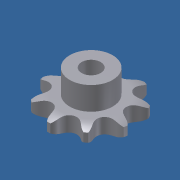
# Autodesk Inventor part: Roller Chain Sprocket1
Saved by Autodesk Inventor 2011 SP1 (Build 150282100, 282)
## iProperties
Created: 2011-02-10
Part Number: Roller Chain Sprocket1
Material: Steel
Document SubType Name: Modeling
Designer: Antonella Wilby
Density: 1 g/cm^3
CustomPartVersion: 1
da_z: 9.0000 ul
da_p: 0.5000 in
da_Dr: 0.3120 in
da_Re: 0.4118 in
da_Ri: 0.1583 in
da_Alfa: 130.00 deg
form_type: 0.0000 ul
da_SC: 0.0023 in
da_Ha: 0.1500 in
da_pt: 0.5660 in
da_k: 1.0000 ul
da_Bf: 0.2962 in
da_Ba: 0.0625 in
da_Rx: 0.5315 in
da_Ra: 0.0200 in
da_Bs: 0.2962 in
da_Ds: 0.8037 in
d42: 0.0000 in
d28: 0.0000 in
d29: 0.0000 in
Author: Antonella Wilby
Autodesk Inventor part; units mm, degrees
ref_plane "YZ Plane" through (0, 0, 0) normal (1, 0, 0) x (0, 1, 0)
ref_plane "XZ Plane" through (0, 0, 0) normal (0, 1, 0) x (-1, 0, 0)
sketch "Theoretical Tooth Profile" plane through (0, 0, 0) normal (0, 0, 1) x (1, 0, 0)
  circle A0 centre (0, 0) radius 18.5662 construction
  line L0 (0, 0) -> (0, 18.5662) construction
  line L1 (0, 0) -> (11.9341, 14.2225) construction
  circle A1 centre (0, 0) radius 21.2565
  arc A2 (-3.0033, 15.8935) -> (3.0033, 15.8935) centre (0, 18.5662) ccw
  line L2 (0, 18.5662) -> (11.9341, 14.2225) construction
  line L3 (0, 18.5662) -> (4.736, 22.7809) construction
  line L4 (4.736, 22.7809) -> (-4.2462, 17.6182) construction
  arc A3 (6.4457, 20.2556) -> (4.5508, 18.1482) centre (10.4256, 14.7715) ccw
  arc A4 (-4.5508, 18.1482) -> (-6.4457, 20.2556) centre (-10.4256, 14.7715) ccw
  line L5 (-10.4256, 14.7715) -> (-4.5508, 18.1482) construction
  arc A5 (-4.2462, 17.6182) -> (-3.0033, 15.8935) centre (4.736, 22.7809) ccw
  line L6 (-4.2462, 17.6182) -> (-4.5508, 18.1482)
  arc A6 (3.0033, 15.8935) -> (4.2462, 17.6182) centre (-4.736, 22.7809) ccw
  line L7 (4.5508, 18.1482) -> (4.2462, 17.6182)
  line L8 (0, 0) -> (7.2701, 19.9746) construction
  point P0 (5.967, 16.3943)
  dimension "d0" = 37.1323
  dimension "d2" = 40
  dimension "d3" = 4.0203
  dimension "d10" = 131.667
  dimension "d11" = 11.778
  dimension "d12" = 6.3398
  dimension "d13" = 10.3602
  dimension "d14" = 11.0947
  dimension "d23" = 3.81
  constraints: 18 end point, 15 point on circle, 7 centre point, 3 coincident, 3 point on line, 3 symmetric about line, 3 tangent, 1 equal radius, 1 midpoint, 1 parallel, 1 vertical, 1 other
  measures "d0" diameter of A0
  measures "d2" angle of L1 L0
  measures "d3" radius of A2
  measures "d10" angle of L3 L0
  measures "d11" angle of L4 L3
  measures "d12" distance of L2.start L3.end
  measures "d13" distance of L3.end L4.end
  measures "d14" distance of A3.centre L0.end
  measures "d23" distance from line of L8.end L2
sketch "Tooth Profile" plane through (0, 0, 0) normal (0, 0, 1) x (1, 0, 0)
  circle A0 centre (0, 0) radius 21.2565 projected
  line L0 (0, 0) -> (0, 18.5662) construction
  line L1 (0, 18.5662) -> (3.6436, 16.8671) construction
  arc A1 (-3.6436, 16.8671) -> (3.6436, 16.8671) centre (0, 18.5662) ccw
  line L2 (-3.6436, 16.8671) -> (0, 18.5662) construction
  arc A2 (-3.6436, 16.8671) -> (-6.238, 20.3206) centre (-13.1243, 12.4462) ccw
  arc A3 (6.238, 20.3206) -> (3.6436, 16.8671) centre (13.1243, 12.4462) ccw
  dimension "d44" = 130
  dimension "d45" = 4.0203
  dimension "d46" = 10.4607
  constraints: 8 point on circle, 7 end point, 3 centre point, 2 tangent, 1 coincident, 1 equal radius, 1 symmetric about line, 1 vertical
  measures "d44" angle of L1 L2
  measures "d45" radius of A1
  measures "d46" radius of A3
sketch "Section Profile" plane through (0, 0, 0) normal (1, 0, 0) x (0, 1, 0)
  line L0 (21.2565, 0) -> (-21.2565, 0) projected
  line L1 (10.2075, 3.7612) -> (-10.2075, 3.7612)
  line L2 (-10.2075, 3.7612) -> (-10.2075, -3.7612)
  line L3 (-10.2075, -3.7612) -> (10.2075, -3.7612)
  line L4 (10.2075, -3.7612) -> (10.2075, 3.7612)
  line L5 (10.2075, 3.7612) -> (21.2565, 3.7612) construction
  line L6 (21.2565, 3.7612) -> (21.2565, -3.7612) construction
  line L7 (21.2565, -3.7612) -> (10.2075, -3.7612) construction
  line L8 (10.2075, -3.7612) -> (10.2075, 3.7612)
  arc A0 (21.2565, 2.1737) -> (14.9049, 3.7612) centre (14.9049, -9.7389) ccw
  arc A1 (14.9049, -3.7612) -> (21.2565, -2.1737) centre (14.9049, 9.7389) ccw
  line L9 (14.9049, 3.7612) -> (0, 3.7612)
  line L10 (0, 3.7612) -> (0, -3.7612)
  line L11 (0, -3.7612) -> (14.9049, -3.7612)
  line L12 (0, 3.7612) -> (0, -3.7612)
  line L13 (21.2565, 2.1737) -> (21.2565, -2.1737)
  point P0 (0, 0)
  point P1 (0, 0)
  dimension "d30" = 7.5225
  dimension "d31" = 20.415
  dimension "d32" = 7.5225
  dimension "d33" = 1.5875
  dimension "d34" = 13.5001
  dimension "d43" = 3.7612
  constraints: 26 end point, 7 midpoint, 5 perpendicular, 4 parallel, 4 point on circle, 3 point on line, 3 symmetric about line, 2 centre point, 2 horizontal, 2 tangent, 1 collinear, 1 other
  measures "d30" distance between parallel lines of L7 L5
  measures "d31" distance between parallel lines of L2 L4
  measures "d32" distance between parallel lines of L3 L1
  measures "d33" distance from line of L13.start L5
  measures "d34" radius of A0
  measures "d43" distance between parallel lines of L3 L0
revolve "Shroud" add sketch "Section Profile" angle 360 about axis through (0, 0, 3.7612) along (0, 0, -1) contours L10 L3 L2 L0 | L0 L2 L1 L10
revolve "Strand" add sketch "Section Profile" angle 360 about axis through (0, 0, 3.7612) along (0, 0, -1) contours L13 A1 L11 L4 L0 | L0 L4 L9 A0 L13 | L4 L3 L10 L0 | L0 L10 L1 L4
pattern_of_one "Strand Pattern"
extrude "Theoretical Tooth" cut sketch "Theoretical Tooth Profile" along normal through all both and the other way through all contours A3 L7 A6 A2 A5 L6 A4 A1 picked at (0.1611, 18.9547)
extrude "Tooth" [suppressed]
pattern_circular "Tooth Pattern" count 9 over 360 about axis through (0, 0, -10) along (0, 0, 1) of "Theoretical Tooth"
ref_plane "Timing Plane" through (0, 18.5662, 0) normal (1, 0, 0) x (0, 1, 0)
sketch "Sketch4" plane through (0, 18.5662, 3.7612) normal (0, 0, 1) x (1, 0, 0)
  arc A0 (14.3472, -14.5273) -> (10.6714, -8.1605) centre (0, -18.5662) ccw projected
  circle A1 centre (0, -18.5662) radius 10.7156
  dimension "d51" = 21.4312
  constraints: 1 centre point, 1 coincident
  measures "d51" diameter of A1
extrude "Extrusion4" add sketch "Sketch4" along normal blind 11.5265
sketch "Sketch5" plane through (0, 18.5662, -3.7612) normal (0, 0, -1) x (-1, 0, 0)
  arc A0 (-1.4862, -3.7355) -> (-8.3945, -6.25) centre (0, -18.5662) ccw projected
  circle A1 centre (0, -18.5662) radius 4.7625
  dimension "d54" = 9.525
  constraints: 1 centre point, 1 coincident
  measures "d54" diameter of A1
extrude "Extrusion5" cut sketch "Sketch5" against normal through all
equation "\"d3\" = 0.5 * da_Dr + da_SC"
equation "\"d12\" = 0.8 * da_Dr"
equation "\"d13\" = 1.3 * da_Dr + da_SC"
equation "\"d14\" = 1.4 * da_Dr"
equation "\"d23\" = da_Ha"
equation "\"d44\" = da_Alfa"
equation "\"d45\" = da_Ri"
equation "\"d46\" = da_Re"
equation "\"d30\" = da_Bf"
equation "\"d31\" = da_Ds"
equation "\"d32\" = da_Bs"
equation "\"d33\" = da_Ba"
equation "\"d34\" = da_Rx"
equation "\"d40\" = da_pt"
equation "\"form_type\" = 0"
equation "\"da_z\" = 9"
equation "\"da_p\" = 12.7"
equation "\"da_Dr\" = 7.9248"
equation "\"da_SC\" = 0.05791"
equation "\"da_Ha\" = 3.81"
equation "\"da_pt\" = 14.3764"
equation "\"da_k\" = 1"
equation "\"da_Bf\" = 7.52246"
equation "\"da_Ba\" = 1.5875"
equation "\"da_Rx\" = 13.5001"
equation "\"da_Ra\" = 0.508"
equation "\"da_Bs\" = 7.52246"
equation "\"da_Ds\" = 20.41496"
equation "\"da_Re\" = 10.46074"
equation "\"da_Ri\" = 4.02031"
equation "\"da_Alfa\" = 130deg"
body "Solid1"
